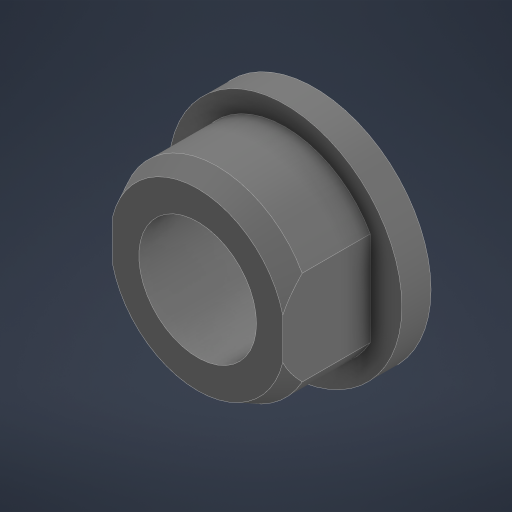
# Autodesk Inventor part: LED-0606
Saved by Autodesk Inventor 2024 (Build 280153000, 153)
## iProperties
Part Number: LED-0606
Material: アセタール樹脂、黒
Document SubType Name: Modeling
Designer: Masato Kubotera
Density: 1.3613 g/cm^3
Appearance: 灰色
Description: ReadyMade
Mass: 0.45 g
Surface Area: 4.68851 cm^2
Volume: 0.330566 cm^3
Catalog Web Link: https://jp.misumi-ec.com/vona2/detail/221000090992/?HissuCode=LED-0606
Author: Masato Kubotera
Autodesk Inventor part; units mm, degrees
ref_plane "YZ Plane" through (0, 0, 0) normal (1, 0, 0) x (0, 1, 0)
ref_plane "XZ Plane" through (0, 0, 0) normal (0, 1, 0) x (-1, 0, 0)
ref_plane "XY Plane" through (0, 0, 0) normal (0, 0, 1) x (1, 0, 0)
sketch "スケッチ1" plane through (0, 0, 0) normal (0, 1, 0) x (-1, 0, 0)
  line L0 (3, 0) -> (6, 0)
  line L1 (6, 0) -> (6, 1.5)
  line L2 (6, 1.5) -> (5, 1.5)
  line L3 (5, 1.5) -> (5, 5)
  line L4 (4.5, 6) -> (3, 6)
  line L5 (3, 6) -> (3, 0)
  line L6 (5, 5) -> (4.5, 6)
  line L7 (0, -1.2) -> (0, 7.2) projected
  point P0 (0, 0)
  point P1 (3, 6)
  dimension "d5" = 1.5
  dimension "d9" = 1
  dimension "d10" = 0.5
  dimension "d17" = 10
  dimension "d18" = 12
  dimension "d19" = 6
  dimension "d20" = 6
  constraints: 14 end point, 4 perpendicular, 1 horizontal, 1 parallel, 1 point on line
  measures "d5" distance of L0.end L1.end
  measures "d9" vertical distance of L3.end L4.start
  measures "d10" horizontal distance of L4.start L3.end
  measures "d17" diameter of L3.end L7
  measures "d18" diameter of L0.end L7
  measures "d19" distance of L4.end L0.start
  measures "d20" diameter of L5 L7
revolve "回転1" add sketch "スケッチ1" angle 360 about axis through (0, 0, -10) along (0, 0, 1)
sketch "スケッチ2" plane through (0, 0, 6) normal (0, 0, 1) x (1, 0, 0)
  line L0 (4.4, -2.3749) -> (-4.4, -2.3749)
  line L1 (-4.4, -2.3749) -> (-4.4, 2.3749)
  line L2 (-4.4, 2.3749) -> (4.4, 2.3749)
  line L3 (4.4, 2.3749) -> (4.4, -2.3749)
  line L4 (4.4, -2.3749) -> (-4.4, 2.3749) construction
  line L5 (-4.4, -2.3749) -> (4.4, 2.3749) construction
  circle A0 centre (0, 0) radius 5
  point P0 (0, 0)
  dimension "d12" = 10
  dimension "d11" = 8.8
  constraints: 12 end point, 2 midpoint, 2 parallel, 1 coincident, 1 horizontal, 1 perpendicular, 3 other
  measures "d11" distance of L1.end L2.end
extrude "押し出し1" cut sketch "スケッチ2" against normal up to surface (4.5 mm away) contours L3 A0 | A0 L1
sketch "스케치3" plane through (0, 0, 6) normal (0, 0, 1) x (1, 0, 0)
  circle A0 centre (0, 0) radius 3 projected
  line L0 (4.4, -0.9434) -> (4.4, 0.9434) projected
  arc A1 (4.4, 0.9434) -> (-4.4, 0.9434) centre (0, 0) ccw projected
  line L1 (-4.4, 0.9434) -> (-4.4, -0.9434) projected
  arc A2 (-4.4, -0.9434) -> (4.4, -0.9434) centre (0, 0) ccw projected
  circle A3 centre (0, 0) radius 3.025
  dimension "d21" = 6.05
  constraints: 1 centre point, 1 coincident
  measures "d21" diameter of A3
extrude "돌출2" cut sketch "스케치3" against normal up to surface (6 mm away) contours A0 | A3
sketch "스케치4" plane through (0, 0, 6) normal (0, 0, 1) x (1, 0, 0)
  circle A0 centre (0, 0) radius 3.025 projected
  line L0 (4.4, -0.9434) -> (4.4, 0.9434) projected
  arc A1 (4.4, 0.9434) -> (-4.4, 0.9434) centre (0, 0) ccw projected
  line L1 (-4.4, 0.9434) -> (-4.4, -0.9434) projected
  arc A2 (-4.4, -0.9434) -> (4.4, -0.9434) centre (0, 0) ccw projected
  line L2 (4.4, 0.9434) -> (4.4, 2.3749) projected
  arc A3 (4.4, 2.3749) -> (-4.4, 2.3749) centre (0, 0) ccw projected
  line L3 (-4.4, 2.3749) -> (-4.4, 0.9434) projected
  arc A4 (4.4, 0.9434) -> (-4.4, 0.9434) centre (0, 0) ccw projected
  line L4 (4.4, -2.3749) -> (4.4, -0.9434) projected
  arc A5 (-4.4, -0.9434) -> (4.4, -0.9434) centre (0, 0) ccw projected
  line L5 (-4.4, -0.9434) -> (-4.4, -2.3749) projected
  arc A6 (-4.4, -2.3749) -> (4.4, -2.3749) centre (0, 0) ccw projected
  arc A7 (4.375, 0.9407) -> (-4.375, 0.9407) centre (0, 0) ccw
  line L6 (4.375, 2.4206) -> (4.375, -2.4206)
  arc A8 (-4.375, -0.9407) -> (4.375, -0.9407) centre (0, 0) ccw
  line L7 (-4.375, -2.4206) -> (-4.375, 2.4206)
  point P0 (-4.35, 2.4653)
  point P1 (-4.35, -2.4653)
  point P2 (4.35, 2.4653)
  point P3 (4.35, -2.4653)
  point P4 (4.4, -0.9434)
  point P5 (4.4, 0.9434)
  point P6 (-4.4, 0.9434)
  point P7 (-4.4, -0.9434)
  point P8 (-4.4, 0.9434)
  point P9 (4.4, 0.9434)
  point P10 (-4.4, -0.9434)
  point P11 (4.4, -0.9434)
  dimension "d27" = 0.025
  constraints: 12 point on circle, 4 end point, 4 point on line, 2 centre point
  measures "d27" radial gap between concentric circles of A1 A7
extrude "돌출3" cut sketch "스케치4" against normal up to surface (4.5 mm away) contours A2 L6 A1 L0 | L4 A6 L6 A2 | A1 L6 A3 L2 | L7 A6 L5 A2 | A2 L1 A1 L7 | A1 L3 A3 L7
